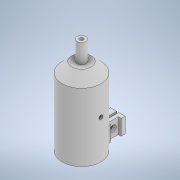
# Autodesk Inventor part: OMEGAETTE_HOUSING
Saved by Autodesk Inventor 2020 (Build 240168000, 168)
## iProperties
Created: 2020-06-15
Part Number: OMEGAETTE_HOUSING
Material: Generic
Document SubType Name: Modeling
Designer: Admin
Density: 1 g/cm^3
Appearance: Default
Author: Admin
Autodesk Inventor part; units mm, degrees
ref_plane "YZ Plane" through (0, 0, 0) normal (1, 0, 0) x (0, 1, 0)
ref_plane "XZ Plane" through (0, 0, 0) normal (0, 1, 0) x (-1, 0, 0)
ref_plane "XY Plane" through (0, 0, 0) normal (0, 0, 1) x (1, 0, 0)
sketch "Sketch1" plane through (0, 0, 0) normal (0, 1, 0) x (-1, 0, 0)
  circle A0 centre (0, 0) radius 10
  dimension "d0" = 20
  constraints: 1 centre point, 1 coincident
  measures "d0" diameter of A0
extrude "Extrusion1" add sketch "Sketch1" along normal blind 40
sketch "Sketch2" plane through (0, 40, 0) normal (0, 1, 0) x (1, 0, 0)
  circle A0 centre (0, 0) radius 2.25
  dimension "d3" = 4.5
  constraints: 1 centre point, 1 coincident
  measures "d3" diameter of A0
extrude "Extrusion2" add sketch "Sketch2" along normal blind 10
sketch "Sketch3" plane through (0, 50, 0) normal (0, 1, 0) x (1, 0, 0)
  circle A0 centre (0, 0) radius 1
  dimension "d6" = 2
  constraints: 1 centre point, 1 coincident
  measures "d6" diameter of A0
extrude "Extrusion3" cut sketch "Sketch3" against normal through all
sketch "Sketch4" plane through (0, 0, 0) normal (0, -1, 0) x (1, 0, 0)
  circle A0 centre (0, 0) radius 7.9
  dimension "d9" = 15.8
  constraints: 1 centre point, 1 coincident
  measures "d9" diameter of A0
extrude "Extrusion4" cut sketch "Sketch4" against normal blind 10
sketch "Sketch5" plane through (0, 10, 0) normal (0, -1, 0) x (1, 0, 0)
  circle A0 centre (0, 0) radius 6.5
  dimension "d12" = 13
  constraints: 1 centre point, 1 coincident
  measures "d12" diameter of A0
extrude "Extrusion5" cut sketch "Sketch5" against normal blind 28
chamfer "Chamfer2" distance 5 angle 45 1 edges at (-6.5, 38, 0)
chamfer "Chamfer3" distance 1.4 angle 45 1 edges at (-6.5, 10, 0)
sketch "Sketch6" plane through (0, 0, 0) normal (0, -1, 0) x (1, 0, 0)
  line L0 (3.75, -9.2702) -> (-3.75, -9.2702)
  line L1 (-3.75, -9.2702) -> (-3.75, -18.7702)
  line L2 (-3.75, -18.7702) -> (3.75, -18.7702)
  line L3 (3.75, -18.7702) -> (3.75, -9.2702)
  circle A0 centre (0, 0) radius 10 projected
  point P0 (-3.75, -9.2702)
  dimension "d24" = 9.5
  dimension "d25" = 7.5
  dimension "d26" = 3.75
  constraints: 8 end point, 2 parallel, 1 horizontal, 1 perpendicular, 2 other
  measures "d24" distance of L2.end L0.start
  measures "d25" distance of L1.end L2.end
  measures "d26" distance from line of point (0, 0) L3
extrude "Extrusion6" add sketch "Sketch6" against normal blind 8 contours L3 L2 L1 A0
sketch "Sketch7" plane through (0, 0, 0) normal (0, -1, 0) x (1, 0, 0)
  line L0 (3.75, -11.2702) -> (2.25, -11.2702)
  line L1 (2.25, -11.2702) -> (2.25, -16.7702)
  line L2 (2.25, -16.7702) -> (3.75, -16.7702)
  line L3 (3.75, -16.7702) -> (3.75, -11.2702)
  line L4 (-3.75, -18.7702) -> (3.75, -18.7702) projected
  line L5 (3.75, -18.7702) -> (3.75, -9.2702) projected
  point P0 (0, 0)
  dimension "d29" = 1.5
  dimension "d30" = 5.5
  dimension "d31" = 2
  constraints: 8 end point, 2 parallel, 1 horizontal, 1 perpendicular, 1 point on line
  measures "d29" distance of L1.end L2.end
  measures "d30" distance of L2.end L0.start
  measures "d31" distance between parallel lines of L4 L2
extrude "Extrusion7" cut sketch "Sketch7" against normal through all
sketch "Sketch8" plane through (0, 0, 0) normal (0, -1, 0) x (1, 0, 0)
  line L0 (-0.5, -18.7702) -> (0.5, -18.7702)
  line L1 (0.5, -18.7702) -> (0.5, -7.8842)
  line L2 (0.5, -7.8842) -> (-0.5, -7.8842)
  line L3 (-0.5, -7.8842) -> (-0.5, -18.7702)
  line L4 (-3.75, -18.7702) -> (3.75, -18.7702) projected
  circle A0 centre (0, 0) radius 7.9 projected
  dimension "d34" = 1
  dimension "d35" = 0.5
  constraints: 8 end point, 2 parallel, 1 horizontal, 1 perpendicular, 1 point on line, 2 other
  measures "d34" distance of L0.start L0.end
  measures "d35" horizontal distance of point (0, 0) L1.end
extrude "Extrusion8" cut sketch "Sketch8" against normal blind 10 contours L3 A0 L1 L0
sketch "Sketch9" plane through (-3.75, 0, -18.7702) normal (-1, 0, 0) x (0, 0, 1)
  circle A0 centre (4.75, 4) radius 1.65
  line L0 (0, 0) -> (0, 8) projected
  line L1 (0, 8) -> (9.5, 8) projected
  point P0 (18.7702, 0)
  dimension "d38" = 3.3
  dimension "d39" = 4.75
  dimension "d40" = 4
  constraints: 1 centre point
  measures "d38" diameter of A0
  measures "d39" distance from line of L0 A0.centre
  measures "d40" distance from line of L1 A0.centre
extrude "Extrusion9" cut sketch "Sketch9" against normal through all
chamfer "Chamfer4" distance 5 angle 45 1 edges at (10, 40, 0)
sketch "Sketch10" plane through (3.75, 0, -18.7702) normal (1, 0, 0) x (0, 0, -1)
  circle A0 centre (-18.7702, 20) radius 1
  line L0 (0, 0) -> (-2, 0) projected
  point P0 (-18.7702, 0)
  dimension "d46" = 2
  dimension "d47" = 20
  dimension "d48" = 0
  constraints: 1 centre point
  measures "d46" diameter of A0
  measures "d47" distance from line of A0.centre L0
  measures "d48" horizontal distance of A0.centre point (-18.77, 0)
extrude "Extrusion10" cut sketch "Sketch10" along normal through all
body "Solid1"
